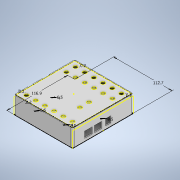
# Autodesk Inventor part: carcasaXeotype1
Saved by Autodesk Inventor 2020 (Build 240168000, 168)
## iProperties
Created: 2021-03-24
Part Number: carcasaXeotype1
Material: Generic
Document SubType Name: Modeling
Designer: Vlasciar
Density: 1 g/cm^3
Appearance: Default
Author: Vlasciar
Autodesk Inventor part; units mm, degrees
ref_plane "YZ Plane" through (0, 0, 0) normal (1, 0, 0) x (0, 1, 0)
ref_plane "XZ Plane" through (0, 0, 0) normal (0, 1, 0) x (-1, 0, 0)
ref_plane "XY Plane" through (0, 0, 0) normal (0, 0, 1) x (1, 0, 0)
sketch "Sketch1" plane through (0, 0, 0) normal (0, 1, 0) x (-1, 0, 0)
  line L0 (-56.35, -58.45) -> (56.35, -58.45)
  line L1 (56.35, -58.45) -> (56.35, 58.45)
  line L2 (56.35, 58.45) -> (-56.35, 58.45)
  line L3 (-56.35, 58.45) -> (-56.35, -58.45)
  line L4 (-56.35, -58.45) -> (56.35, 58.45) construction
  line L5 (56.35, -58.45) -> (-56.35, 58.45) construction
  point P0 (0, 0)
  dimension "d0" = 116.9
  dimension "d1" = 112.7
  constraints: 12 end point, 2 midpoint, 2 parallel, 1 horizontal, 1 perpendicular
  measures "d0" distance between parallel lines of L0 L2
  measures "d1" distance between parallel lines of L3 L1
extrude "Extrusion1" add sketch "Sketch1" along normal blind 29.55
sketch "Sketch2" plane through (56.35, 0, 58.45) normal (1, 0, 0) x (0, 0, -1)
  line L0 (0, 0) -> (116.9, 0) projected
  line L1 (116.9, 0) -> (116.9, 29.55) projected
  line L2 (0, 29.55) -> (116.9, 29.55) projected
  line L3 (0, 0) -> (0, 29.55) projected
  point P0 (58.45, 0)
shell "Shell1" thickness 2 removed faces 1 at (18.7833, 29.55, -19.4833)
sketch "Sketch3" plane through (56.35, 0, 58.45) normal (1, 0, 0) x (0, 0, -1)
  line L0 (0, 0) -> (116.9, 0) projected
  line L1 (116.9, 0) -> (116.9, 29.55) projected
  line L2 (0, 0) -> (0, 29.55) projected
  line L3 (114.9, 29.55) -> (2, 29.55) projected
  line L4 (1.5, 29.55) -> (1.5, 0)
  line L5 (114.9, 29.55) -> (114.9, 0)
  line L6 (37.75, 15.2) -> (37.75, 3.2)
  line L7 (23.4, 15.2) -> (23.4, 3)
  line L8 (114.9, 2) -> (114.9, 29.55) projected
  line L9 (56, 15.2) -> (56, 3.2)
  line L10 (42.1, 15.2) -> (42.1, 3.2)
  line L11 (63.75, 15.7) -> (63.75, 3.7)
  line L12 (73.55, 15.7) -> (73.55, 3.7)
  line L13 (0, 3.2) -> (1.5, 3.2)
  line L14 (23.4, 3.2) -> (37.75, 3.2)
  line L15 (23.4, 15.2) -> (37.75, 15.2)
  line L16 (42.1, 15.2) -> (56, 15.2)
  line L17 (63.75, 15.7) -> (73.55, 15.7)
  line L18 (42.1, 3.2) -> (56, 3.2)
  line L19 (63.75, 3.7) -> (73.55, 3.7)
  line L20 (114.9, 3.7) -> (116.9, 3.7)
  point P0 (58.45, 0)
  dimension "d6" = 1.5
  dimension "d7" = 2
  dimension "d8" = 36.25
  dimension "d9" = 21.9
  dimension "d10" = 14.35
  dimension "d12" = 54.5
  dimension "d13" = 40.6
  dimension "d14" = 13.9
  dimension "d15" = 51.15
  dimension "d16" = 41.35
  dimension "d17" = 9.8
  constraints: 32 end point, 30 perpendicular, 8 point on line, 3 horizontal, 3 vertical
  measures "d6" distance between parallel lines of L4 L2
  measures "d7" distance between parallel lines of L5 L1
  measures "d8" distance between parallel lines of L6 L4
  measures "d9" distance between parallel lines of L4 L7
  measures "d10" distance between parallel lines of L6 L7
  measures "d12" distance between parallel lines of L4 L9
  measures "d13" distance between parallel lines of L4 L10
  measures "d14" distance between parallel lines of L9 L10
  measures "d15" distance between parallel lines of L8 L11
  measures "d16" distance between parallel lines of L8 L12
  measures "d17" distance between parallel lines of L12 L11
sketch "Sketch4" plane through (56.35, 0, 58.45) normal (1, 0, 0) x (0, 0, -1)
  line L0 (0, 0) -> (116.9, 0) projected
  line L1 (116.9, 0) -> (116.9, 29.55) projected
  line L2 (0, 29.55) -> (116.9, 29.55) projected
  line L3 (0, 0) -> (0, 29.55) projected
  point P0 (58.45, 0)
extrude "Extrusion2" cut sketch "Sketch3" against normal blind 29.55 contours L6 L14 L7 L15 | L9 L18 L10 L16 | L17 L12 L19 L11
sketch "Sketch5" plane through (-54.35, 2, -56.45) normal (0, 1, 0) x (1, 0, 0)
  line L0 (108.7, -112.9) -> (108.7, 0) projected
  line L1 (108.7, 0) -> (0, 0) projected
  line L2 (0, 0) -> (0, -112.9) projected
  line L3 (0, -112.9) -> (108.7, -112.9) projected
  point P0 (54.35, -56.45)
sketch "Sketch6" plane through (-56.35, 0, -58.45) normal (-1, 0, 0) x (0, 0, 1)
  line L0 (0, 0) -> (116.9, 0) projected
  line L1 (116.9, 0) -> (116.9, 29.55) projected
  line L2 (0, 29.55) -> (116.9, 29.55) projected
  line L3 (0, 0) -> (0, 29.55) projected
  point P0 (58.45, 0)
sketch "Sketch7" plane through (-56.35, 0, -58.45) normal (-1, 0, 0) x (0, 0, 1)
  line L0 (116.9, 0) -> (116.9, 29.55) projected
  line L1 (0, 29.55) -> (116.9, 29.55) projected
  line L2 (0, 0) -> (0, 29.55) projected
  line L3 (116.9, 0) -> (116.9, 29.55) projected
  line L4 (94.4, 13.85) -> (94.4, 29.55)
  line L5 (114.9, 2) -> (114.9, 29.55) projected
  line L6 (40.65, 29.55) -> (40.65, 13.85)
  line L7 (2, 2) -> (2, 29.55) projected
  line L8 (0, 13.85) -> (2, 13.85)
  line L9 (40.65, 13.85) -> (94.4, 13.85)
  line L10 (114.9, 14.35) -> (116.9, 14.35)
  line L11 (0, 3.2) -> (2, 3.2)
  line L12 (114.9, 3.7) -> (116.9, 3.7)
  point P0 (58.45, 0)
  dimension "d22" = 20.5
  dimension "d23" = 74.25
  dimension "d24" = 38.65
  constraints: 14 end point, 10 point on line, 9 perpendicular
  measures "d22" distance between parallel lines of L5 L4
  measures "d23" distance between parallel lines of L5 L6
  measures "d24" distance between parallel lines of L7 L6
extrude "Extrusion3" cut sketch "Sketch7" against normal blind 29.55 fills toward (40.7, 21.7) open curves L6 L9 L4
sketch "Sketch8" plane through (-54.35, 2, -56.45) normal (0, 1, 0) x (1, 0, 0)
  line L0 (108.7, -112.9) -> (108.7, 0) projected
  line L1 (108.7, 0) -> (0, 0) projected
  line L2 (0, 0) -> (0, -112.9) projected
  line L3 (0, -112.9) -> (108.7, -112.9) projected
  point P0 (54.35, -56.45)
sketch "Sketch9" plane through (0, 0, 0) normal (0, -1, 0) x (1, 0, 0)
  line L0 (56.35, 58.45) -> (56.35, -58.45) projected
  line L1 (-56.35, 58.45) -> (56.35, 58.45) projected
  line L2 (-56.35, -58.45) -> (-56.35, 58.45) projected
  line L3 (56.35, -58.45) -> (-56.35, -58.45) projected
  line L4 (-54.55, -56.65) -> (54.55, -56.65)
  line L5 (54.55, -56.65) -> (54.55, 56.65)
  line L6 (54.55, 56.65) -> (-54.55, 56.65)
  line L7 (-54.55, 56.65) -> (-54.55, -56.65)
  point P0 (0, 0)
  dimension "d28" = 1.8
  dimension "d29" = 1.8
  dimension "d30" = 1.8
  dimension "d31" = 1.8
  constraints: 8 end point, 2 parallel, 1 horizontal, 1 perpendicular
  measures "d28" distance from line of L3 L4.start
  measures "d29" distance from line of L2 L4.start
  measures "d30" distance from line of L1 L5.end
  measures "d31" distance from line of L0 L5.end
extrude "Extrusion4" add sketch "Sketch9" against normal blind 29.55 separate body contours L7 L6 L5 L4
sketch "Sketch10" plane through (-54.55, 0, -56.65) normal (-1, 0, 0) x (0, 0, 1)
  line L0 (113.3, 0) -> (0, 0) projected
  line L1 (113.3, 0) -> (113.3, 29.55) projected
  line L2 (0, 29.55) -> (113.3, 29.55) projected
  line L3 (0, 0) -> (0, 29.55) projected
  line L4 (0, 28.05) -> (113.3, 28.05)
  point P0 (56.65, 0)
  dimension "d34" = 1.5
  constraints: 2 end point, 2 point on line, 1 perpendicular
  measures "d34" distance between parallel lines of L2 L4
extrude "Extrusion5" cut sketch "Sketch10" against normal through all contours L0 L3 L4 L1 bodies 2
sketch "Sketch11" plane through (0, 29.55, 0) normal (0, 1, 0) x (1, 0, 0)
  line L0 (54.55, 56.65) -> (-54.55, 56.65) projected
  line L1 (-54.55, 56.65) -> (-54.55, -56.65) projected
  line L2 (-54.55, -56.65) -> (54.55, -56.65) projected
  line L3 (54.55, -56.65) -> (54.55, 56.65) projected
  line L4 (47.75, 56.65) -> (47.75, -56.65)
  line L5 (-47.75, 56.65) -> (-47.75, -56.65)
  line L6 (-47.75, 50.1) -> (47.75, 50.1)
  line L7 (47.75, -50.1) -> (-47.75, -50.1)
  line L8 (27.05, 29.7) -> (27.05, -47.1)
  point P0 (0, 0)
  point P1 (-44.75, -47.1)
  point P2 (44.75, -47.1)
  point P3 (9.35, -47.1)
  point P4 (-8.35, -47.1)
  point P5 (-26.05, -47.1)
  point P6 (-43.75, -47.1)
  point P7 (44.75, 47.1)
  point P8 (27.05, 47.1)
  point P9 (9.35, 47.1)
  point P10 (-8.35, 47.1)
  point P11 (-26.05, 47.1)
  point P12 (-43.75, 47.1)
  point P13 (44.75, 29.7)
  point P14 (9.35, 29.7)
  point P15 (-8.35, 29.7)
  point P16 (-26.05, 29.7)
  point P17 (-43.75, 29.7)
  point P18 (28.2, 1.2)
  point P19 (28.2, -16.2)
  dimension "d37" = 109.1
  dimension "d38" = 113.3
  dimension "d39" = 6.8
  dimension "d40" = 6.8
  dimension "d41" = 6.55
  dimension "d42" = 6.55
  dimension "d43" = 3
  dimension "d44" = 3
  dimension "d45" = 3
  dimension "d46" = 3
  dimension "d47" = 89.5
  dimension "d50" = 17.7
  dimension "d55" = 3
  dimension "d56" = 3
  dimension "d59" = 17.7
  dimension "d64" = 3
  dimension "d65" = 17.4
  dimension "d68" = 17.7
  dimension "d73" = 1.15
  dimension "d74" = 28.5
  dimension "d75" = 17.4
  dimension "d76" = 30.9
  constraints: 10 end point, 8 point on line, 4 parallel, 3 horizontal, 3 perpendicular, 1 vertical, 1 vertical alignment, 15 other
  measures "d37" distance between parallel lines of L1 L3
  measures "d38" distance between parallel lines of L2 L0
  measures "d39" distance between parallel lines of L3 L4
  measures "d40" distance between parallel lines of L5 L1
  measures "d41" distance between parallel lines of L6 L0
  measures "d42" distance between parallel lines of L7 L2
  measures "d43" distance from line of L5 point (-44.75, -47.1)
  measures "d44" distance from line of L7 point (-44.75, -47.1)
  measures "d45" distance from line of L4 point (44.75, -47.1)
  measures "d46" distance from line of L7 point (44.75, -47.1)
  measures "d47" distance of point (-44.75, -47.1) point (44.75, -47.1)
  measures "d50" distance of point (44.75, -47.1) L8.end
  measures "d55" distance from line of L4 point (44.75, 47.1)
  measures "d56" distance from line of L6 point (44.75, 47.1)
  measures "d59" distance of point (44.75, 47.1) point (27.05, 47.1)
  measures "d64" distance from line of L4 point (44.75, 29.7)
  measures "d65" distance of point (44.75, 47.1) point (44.75, 29.7)
  measures "d68" distance of point (44.75, 29.7) L8.start
  measures "d73" distance from line of L8 point (28.2, 1.2)
  measures "d74" vertical distance of L8.start point (28.2, 1.2)
  measures "d75" distance of point (28.2, -16.2) point (28.2, 1.2)
  measures "d76" vertical distance of L8.end point (28.2, -16.2)
hole "Hole1" at (-43.75, 29.55, -47.1) at (-43.75, 29.55, -29.7) at (-26.05, 29.55, -47.1) at (-26.05, 29.55, -29.7) at (-8.35, 29.55, -47.1) at (-8.35, 29.55, -29.7) at (9.35, 29.55, -47.1) at (9.35, 29.55, -29.7) at (27.05, 29.55, -47.1) at (27.05, 29.55, -29.7) at (44.75, 29.55, -47.1) at (44.75, 29.55, -29.7) direction (0, -1, 0) diameter 7 end through all bodies 2
hole "Hole2" at (44.75, 29.55, 47.1) at (9.35, 29.55, 47.1) at (-8.35, 29.55, 47.1) at (-26.05, 29.55, 47.1) at (-43.75, 29.55, 47.1) at (27.05, 29.55, 47.1) direction (0, -1, 0) diameter 7 end through all bodies 2
hole "Hole3" at (28.2, 29.55, 16.2) at (28.2, 29.55, -1.2) direction (0, -1, 0) diameter 7 end through all bodies 2
sketch "Sketch13" plane through (-54.55, 29.55, -56.65) normal (-1, 0, 0) x (0, 0, 1)
  line L0 (0, -1.5) -> (113.3, -1.5) projected
  line L1 (35, -1.5) -> (35, -17) projected
  line L2 (95, -17) -> (35, -17) projected
  line L3 (95, -1.5) -> (95, -17) projected
  line L4 (0, -1.5) -> (113.3, -1.5) projected
  line L5 (113.3, -1.5) -> (113.3, 0) projected
  line L6 (0, 0) -> (113.3, 0) projected
  line L7 (0, -1.5) -> (0, 0) projected
  line L8 (113.3, 0) -> (0, 0) projected
  line L9 (0.15, 0) -> (0.15, -1.5)
  line L10 (113.15, 0) -> (113.15, -1.5)
  line L11 (47.65, -1.5) -> (47.65, -17)
  line L12 (60.75, -1.5) -> (60.75, -17)
  line L13 (35, -1.5) -> (35, -17) projected
  line L14 (76.35, -1.5) -> (69.35, -1.5) projected
  line L15 (79.15, -1.5) -> (79.15, -17)
  line L16 (35, -17) -> (95, -17) projected
  line L17 (113.3, -1.5) -> (0, -1.5) projected
  line L18 (89.15, -1.5) -> (89.15, -17)
  line L19 (47.65, -1.5) -> (60.75, -1.5)
  line L20 (79.15, -1.5) -> (89.15, -1.5)
  line L21 (38.85, -15.7) -> (38.85, 0) projected
  line L22 (92.6, 0) -> (92.6, -15.7) projected
  point P0 (56.65, -29.55)
  dimension "d101" = 0.15
  dimension "d102" = 0.15
  dimension "d103" = 113
  dimension "d104" = 65.5
  dimension "d105" = 13.1
  dimension "d106" = 34
  dimension "d107" = 10
  dimension "d108" = 8.8
  dimension "d109" = 3.45
  dimension "d110" = 18.4
  constraints: 16 end point, 9 point on line, 5 perpendicular, 2 vertical, 1 parallel, 2 other
  measures "d101" distance between parallel lines of L7 L9
  measures "d102" distance between parallel lines of L5 L10
  measures "d103" distance between parallel lines of L9 L10
  measures "d104" distance between parallel lines of L11 L10
  measures "d105" distance between parallel lines of L12 L11
  measures "d106" distance between parallel lines of L15 L10
  measures "d107" distance between parallel lines of L18 L15
  measures "d108" distance between parallel lines of L11 L21
  measures "d109" distance between parallel lines of L22 L18
  measures "d110" distance between parallel lines of L12 L15
sketch "Sketch14" plane through (-56.35, 13.85, 35.95) normal (0, 1, 0) x (1, 0, 0)
  line L0 (2, 53.75) -> (2, 0) projected
  line L1 (0, 53.75) -> (2, 53.75) projected
  line L2 (0, 0) -> (0, 53.75) projected
  line L3 (0, 0) -> (2, 0) projected
  line L4 (2, 45.45) -> (0, 45.45)
  line L5 (2, 32.35) -> (0, 32.35)
  line L6 (2, 92.4) -> (2, -20.5) projected
  line L7 (2, 3.95) -> (0, 3.95)
  line L8 (2, 13.95) -> (0, 13.95)
  point P0 (56.35, 35.95)
  point P1 (2, 3.95)
  point P2 (2, 13.95)
  dimension "d111" = 8.3
  dimension "d112" = 13.1
  dimension "d113" = 18.4
  dimension "d114" = 10
  constraints: 8 end point, 8 point on line, 2 parallel, 2 perpendicular
  measures "d111" distance between parallel lines of L4 L1
  measures "d112" distance between parallel lines of L5 L4
  measures "d113" distance between parallel lines of L5 L8
  measures "d114" distance between parallel lines of L8 L7
extrude "Extrusion7" add sketch "Sketch14" along normal blind 15.7 contours L0 L4 L2 L1 | L0 L8 L2 L5 | L0 L3 L2 L7 bodies 1
sketch "Sketch15" plane through (-56.35, 13.85, 3.6) normal (0, 1, 0) x (1, 0, 0)
  line L0 (0, 0) -> (2, 0) projected
  line L1 (2, 13.1) -> (2, 0) projected
  line L2 (2, 13.1) -> (0, 13.1) projected
  line L3 (0, 0) -> (0, 13.1) projected
  point P0 (56.35, 3.6)
extrude "Extrusion8" add sketch "Sketch15" along normal blind 2 bodies 1
sketch "Sketch16" plane through (-56.35, 13.85, 32) normal (0, 1, 0) x (1, 0, 0)
  line L0 (0, 0) -> (2, 0) projected
  line L1 (2, 10) -> (2, 0) projected
  line L2 (2, 10) -> (0, 10) projected
  line L3 (0, 0) -> (0, 10) projected
  point P0 (56.35, 32)
extrude "Extrusion9" add sketch "Sketch16" along normal blind 2 bodies 1
extrude "Extrusion10" add sketch "Sketch1" against normal blind 1.75 bodies 1
extrude "Extrusion11" cut sketch "Sketch5" against normal blind 1.75 bodies 1
move or copy body "Move Body4" bodies to move or copy 1 copy no translate (0, 1.75, 0)
fillet "Fillet1" radius 3.5 4 edges at (-56.35, 15.65, -58.45) (56.35, 15.65, -58.45) (-56.35, 15.65, 58.45) (56.35, 15.65, 58.45)
sketch "Sketch17" plane through (-54.35, 2, -56.45) normal (0, 1, 0) x (1, 0, 0)
  circle A0 centre (16, -88.9) radius 2
  circle A1 centre (9.6, -50.7) radius 2
  circle A2 centre (9.6, -50.7) radius 3.25
  circle A3 centre (16, -88.9) radius 3.25
  line L0 (108.7, -112.9) -> (0, -112.9) projected
  circle A4 centre (67.1, -84.4) radius 2
  circle A5 centre (67.1, -84.4) radius 3.25
  circle A6 centre (92.4, -38.3) radius 2
  circle A7 centre (92.4, -38.3) radius 3.25
  point P0 (54.35, -56.45)
  dimension "d145" = 4
  dimension "d146" = 4
  dimension "d147" = 6.5
  dimension "d148" = 6.5
  dimension "d161" = 4
  dimension "d162" = 6.5
  dimension "d163" = 4
  dimension "d164" = 6.5
  constraints: 9 coincident, 8 centre point
  measures "d145" diameter of A0
  measures "d146" diameter of A1
  measures "d147" diameter of A2
  measures "d148" diameter of A3
  measures "d161" diameter of A4
  measures "d162" diameter of A5
  measures "d163" diameter of A6
  measures "d164" diameter of A7
extrude "Extrusion12" add sketch "Sketch17" along normal blind 3 contours A2 | A3 bodies 1
extrude "Extrusion13" cut sketch "Sketch17" against normal blind 3 contours A0 | A1 bodies 1
extrude "Extrusion14" add sketch "Sketch17" along normal blind 3 contours A5 | A7 bodies 1
extrude "Extrusion15" cut sketch "Sketch17" against normal blind 3 contours A4 | A6 bodies 1
move or copy body "Move Body5" bodies to move or copy 2 copy no translate (0, 3.25, 0)
sketch "Sketch19" plane through (-54.35, 31.3, -56.45) normal (0, 1, 0) x (1, 0, 0)
  arc A0 (107.2, -114.9) -> (110.7, -111.4) centre (107.2, -111.4) ccw projected
  line L0 (110.7, -111.4) -> (110.7, -1.5) projected
  arc A1 (110.7, -1.5) -> (107.2, 2) centre (107.2, -1.5) ccw projected
  line L1 (107.2, 2) -> (1.5, 2) projected
  arc A2 (1.5, 2) -> (-2, -1.5) centre (1.5, -1.5) ccw projected
  line L2 (-2, -1.5) -> (-2, -46.95) projected
  line L3 (-2, -46.95) -> (0, -46.95) projected
  line L4 (0, -46.95) -> (0, 0) projected
  line L5 (0, 0) -> (108.7, 0) projected
  line L6 (108.7, 0) -> (108.7, -112.9) projected
  line L7 (108.7, -112.9) -> (0, -112.9) projected
  line L8 (0, -112.9) -> (0, -88.45) projected
  line L9 (0, -88.45) -> (-2, -88.45) projected
  line L10 (-2, -88.45) -> (-2, -111.4) projected
  arc A3 (-2, -111.4) -> (1.5, -114.9) centre (1.5, -111.4) ccw projected
  line L11 (1.5, -114.9) -> (107.2, -114.9) projected
  point P0 (54.35, -56.45)
extrude "Extrusion17" add sketch "Sketch19" along normal blind 1.5 bodies 1
sketch "Sketch20" plane through (-56.35, 31.3, 3.6) normal (0, 1, 0) x (1, 0, 0)
  line L0 (2, -18.4) -> (2, 0) projected
  line L1 (2, 0) -> (0, 0) projected
  line L2 (0, 0) -> (0, -18.4) projected
  line L3 (0, -18.4) -> (2, -18.4) projected
  point P0 (56.35, 3.6)
extrude "Extrusion18" add sketch "Sketch20" along normal blind 1.5 bodies 1
sketch "Sketch21" plane through (-54.55, 32.8, 56.65) normal (0, 1, 0) x (1, 0, 0)
  circle A0 centre (82.75, 40.45) radius 3.5 projected
  circle A1 centre (82.75, 57.85) radius 3.5 projected
  circle A2 centre (10.8, 9.55) radius 3.5 projected
  circle A3 centre (46.2, 9.55) radius 3.5 projected
  circle A4 centre (99.3, 9.55) radius 3.5 projected
  circle A5 centre (63.9, 9.55) radius 3.5 projected
  circle A6 centre (28.5, 9.55) radius 3.5 projected
  circle A7 centre (81.6, 9.55) radius 3.5 projected
  circle A8 centre (99.3, 103.75) radius 3.5 projected
  circle A9 centre (81.6, 103.75) radius 3.5 projected
  circle A10 centre (63.9, 103.75) radius 3.5 projected
  circle A11 centre (46.2, 103.75) radius 3.5 projected
  circle A12 centre (28.5, 103.75) radius 3.5 projected
  circle A13 centre (10.8, 103.75) radius 3.5 projected
  circle A14 centre (10.8, 86.35) radius 3.5 projected
  circle A15 centre (28.5, 86.35) radius 3.5 projected
  circle A16 centre (46.2, 86.35) radius 3.5 projected
  circle A17 centre (63.9, 86.35) radius 3.5 projected
  circle A18 centre (81.6, 86.35) radius 3.5 projected
  circle A19 centre (99.3, 86.35) radius 3.5 projected
  line L0 (0, 0) -> (109.1, 0) projected
  line L1 (109.1, 0) -> (109.1, 113.3) projected
  line L2 (109.1, 113.3) -> (0, 113.3) projected
  line L3 (0, 113.3) -> (0, 0) projected
  line L4 (109.3, 113.5) -> (-0.2, 113.5)
  line L5 (-0.2, 113.5) -> (-0.2, -0.2)
  line L6 (-0.2, -0.2) -> (109.3, -0.2)
  line L7 (109.3, -0.2) -> (109.3, 113.5)
  point P0 (54.55, 56.65)
  dimension "d182" = 0.2
  dimension "d183" = 0.2
  dimension "d184" = 0.2
  dimension "d185" = 0.2
  constraints: 8 end point, 2 parallel, 1 horizontal, 1 perpendicular
  measures "d182" distance between parallel lines of L6 L0
  measures "d183" distance between parallel lines of L3 L5
  measures "d184" distance between parallel lines of L4 L2
  measures "d185" distance between parallel lines of L7 L1
combine bodies "Combine1" operation type add bodies to combine 1 2
extrude "Extrusion19" add sketch "Sketch17" against normal blind 2 contours A0 | A1 | A4 | A6 bodies 1
body "Solid1"
